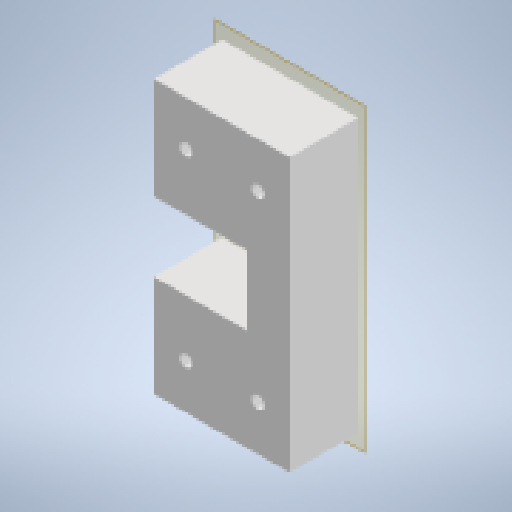
# Autodesk Inventor part: holder1
Saved by Autodesk Inventor 2024 (Build 280153000, 153)
## iProperties
Created: 2023-12-14
Part Number: holder1
Material: Generic
Document SubType Name: Modeling
Designer: Abdulrahman Riskuwa
Density: 1 g/cm^3
Appearance: Default
Author: Abdulrahman Riskuwa
Autodesk Inventor part; units mm, degrees
ref_plane "YZ Plane" through (0, 0, 0) normal (1, 0, 0) x (0, 1, 0)
ref_plane "XZ Plane" through (0, 0, 0) normal (0, 1, 0) x (-1, 0, 0)
ref_plane "XY Plane" through (0, 0, 0) normal (0, 0, 1) x (1, 0, 0)
ref_plane "Work Plane1" through (0, 0, 0) normal (0, 0, 1) x (1, 0, 0)
sketch "Sketch1" plane through (0, 0, 0) normal (0, 0, 1) x (1, 0, 0)
  line L0 (-9.25, 7.625) -> (-9.25, -7.625) projected
  line L1 (-9.25, -7.625) -> (-29.75, -7.625) projected
  line L2 (-29.75, -7.625) -> (-29.75, -29.875) projected
  line L3 (-29.75, -29.875) -> (0, -29.875) projected
  line L4 (0, -29.875) -> (0, 29.875) projected
  line L5 (0, 29.875) -> (-29.75, 29.875) projected
  line L6 (-29.75, 29.875) -> (-29.75, 7.625) projected
  line L7 (-29.75, 7.625) -> (-9.25, 7.625) projected
  circle A0 centre (-15, 14.875) radius 3.5 projected
  circle A1 centre (-15, -14.875) radius 3.5 projected
  circle A2 centre (-7, 20) radius 1.35 projected
  circle A3 centre (-6, 0) radius 1.35 projected
  circle A4 centre (-7, -20) radius 1.35 projected
  circle A5 centre (-22.75, -20) radius 1.35 projected
  circle A6 centre (-22.75, 20) radius 1.35 projected
  line L8 (-29.75, -29.875) -> (0, -29.875)
  line L9 (0, 29.875) -> (-29.75, 29.875)
  point P0 (0, 0)
  constraints: 4 end point, 1 collinear, 1 horizontal
extrude "Extrusion1" add sketch "Sketch1" along normal blind 25.2 contours L7 L6 L5 L4 L3 L2 L1 L0 | A0 | A1 | A3
sketch "Sketch3" plane through (0, -29.875, 0) normal (1, 0, 0) x (0, 0, -1)
  circle A0 centre (-12.6232, 29.875) radius 1.621 projected
  point P0 (0, 29.875)
  constraints: 1 coincident
hole "Hole2" at (0, 0, 12.6232) direction (-1, 0, 0) diameter 3.242 depth 6 thread size "M4x0.7" class "6H" standard "ISO Metric profile"
body "Solid1"
